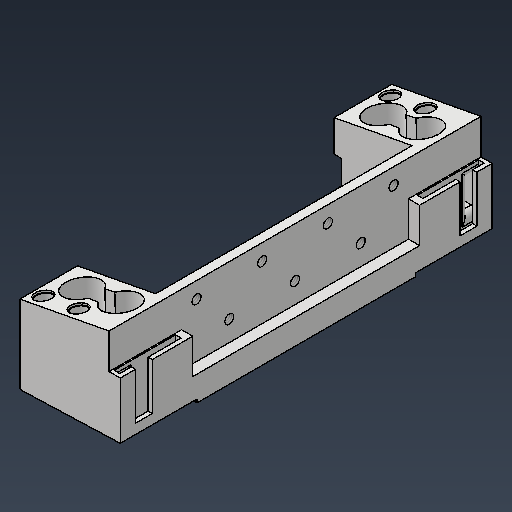
# Autodesk Inventor part: FonrtMount
Saved by Autodesk Inventor 2026.2 (Build 302298010, 298A)
## iProperties
Created: 2026-04-04
Part Number: FonrtMount
Material: Generic
Document SubType Name: Sheet Metal
Designer: szymo
Density: 1 g/cm^3
Appearance: Default
Mass: 17.9089 g
Surface Area: 155.221 cm^2
Volume: 17.9089 cm^3
Sheet Metal Rule: Default
Author: szymo
Autodesk Inventor part; units mm, degrees
(part 1 of 2)
ref_plane "YZ Plane" through (0, 0, 0) normal (1, 0, 0) x (0, 1, 0)
ref_plane "XZ Plane" through (0, 0, 0) normal (0, 1, 0) x (-1, 0, 0)
ref_plane "XY Plane" through (0, 0, 0) normal (0, 0, 1) x (1, 0, 0)
sketch "Sketch1" plane through (0, 0, 0) normal (0, 0, 1) x (1, 0, 0)
  line L0 (-27, 86.2958) -> (-6.5, 86.2958) projected
  line L1 (-6.5, 86.2958) -> (-6.5, 69.7958) projected
  line L2 (-27, 69.7958) -> (-6.5, 69.7958) projected
  line L3 (-27, 86.2958) -> (-27, 69.7958) projected
  line L4 (0, 97) -> (0, 81.9) projected
  line L5 (0, 81.9) -> (-2, 81.9) projected
  line L6 (-4, 93) -> (0, 97) projected
  circle A0 centre (-14.5, 55.2958) radius 14.5 projected
  line L7 (-5.9811, 90.2856) -> (-6, 90.2856)
  line L8 (-6, 90.2856) -> (-6, 69.2958)
  line L9 (-6, 69.2958) -> (-10.7251, 69.2958)
  line L10 (-4, 65.2958) -> (0, 65.2958)
  line L11 (0, 65.2958) -> (0, 81.4)
  line L12 (0, 81.4) -> (-3, 81.4)
  line L13 (-3, 81.4) -> (-3, 90.8556)
  line L14 (-6, 90.2856) -> (-5.9811, 90.2856)
  line L15 (-6, 90.2856) -> (-3, 90.8556)
  line L16 (-9.2085, 69.2958) -> (-9.2085, 68.7958)
  arc A1 (-5.2144, 40.6176) -> (-6.571, 40.1714) centre (-4.0302, 34.7325) ccw construction
  arc A2 (-4.9311, 40.2025) -> (-5.2144, 40.6176) centre (-13, 35.0012) ccw construction
  arc A3 (-5.8414, 39.102) -> (-4.9311, 40.2025) centre (-9.9791, 43.4512) ccw construction
  arc A4 (-5.6366, 38.7217) -> (-5.8414, 39.102) centre (-13, 35.0012) ccw construction
  arc A5 (-4.2168, 38.8762) -> (-5.6366, 38.7217) centre (-4.2821, 32.8735) ccw construction
  arc A6 (-4.026, 38.4112) -> (-4.2168, 38.8762) centre (-13, 35.0012) ccw construction
  arc A7 (-5.1452, 37.524) -> (-4.026, 38.4112) centre (-8.2882, 42.6385) ccw construction
  arc A8 (-5.0239, 37.1095) -> (-5.1452, 37.524) centre (-13, 35.0012) ccw construction
  arc A9 (-3.6031, 36.9654) -> (-5.0239, 37.1095) centre (-4.915, 31.1074) ccw construction
  arc A10 (-3.5132, 36.4709) -> (-3.6031, 36.9654) centre (-13, 35.0012) ccw construction
  arc A11 (-4.7923, 35.8358) -> (-3.5132, 36.4709) centre (-6.8033, 41.492) ccw construction
  arc A12 (-4.7599, 35.4051) -> (-4.7923, 35.8358) centre (-13, 35.0012) ccw construction
  arc A13 (-3.4001, 34.9687) -> (-4.7599, 35.4051) centre (-5.9012, 29.5115) ccw construction
  arc A14 (-3.4149, 34.4663) -> (-3.4001, 34.9687) centre (-13, 35.0012) ccw construction
  arc A15 (-4.7982, 34.1111) -> (-3.4149, 34.4663) centre (-5.5892, 40.0618) ccw construction
  arc A16 (-4.856, 33.6831) -> (-4.7982, 34.1111) centre (-13, 35.0012) ccw construction
  arc A17 (-3.6166, 32.9735) -> (-4.856, 33.6831) centre (-7.1977, 28.1556) ccw construction
  arc A18 (-3.7356, 32.4852) -> (-3.6166, 32.9735) centre (-13, 35.0012) ccw construction
  arc A19 (-5.1625, 32.4253) -> (-3.7356, 32.4852) centre (-4.699, 38.4104) ccw construction
  arc A20 (-5.308, 32.0186) -> (-5.1625, 32.4253) centre (-13, 35.0012) ccw construction
  arc A21 (-4.2432, 31.0669) -> (-5.308, 32.0186) centre (-8.7478, 27.0988) ccw construction
  arc A22 (-4.4611, 30.614) -> (-4.2432, 31.0669) centre (-13, 35.0012) ccw construction
  arc A23 (-5.8693, 30.8521) -> (-4.4611, 30.614) centre (-4.1716, 36.61) ccw construction
  arc A24 (-6.0962, 30.4845) -> (-5.8693, 30.8521) centre (-13, 35.0012) ccw construction
  arc A25 (-5.2526, 29.3322) -> (-6.0962, 30.4845) centre (-10.4837, 26.3874) ccw construction
  arc A26 (-5.5599, 28.9345) -> (-5.2526, 29.3322) centre (-13, 35.0012) ccw construction
  arc A27 (-6.8878, 29.4602) -> (-5.5599, 28.9345) centre (-4.03, 34.7394) ccw construction
  arc A28 (-7.1861, 29.1479) -> (-6.8878, 29.4602) centre (-13, 35.0012) ccw construction
  arc A29 (-6.6005, 27.8453) -> (-7.1861, 29.1479) centre (-12.3296, 26.0525) ccw construction
  arc A30 (-6.9838, 27.5202) -> (-6.6005, 27.8453) centre (-13, 35.0012) ccw construction
  arc A31 (-8.1734, 28.3104) -> (-6.9838, 27.5202) centre (-4.2805, 32.8801) ccw construction
  arc A32 (-8.5302, 28.067) -> (-8.1734, 28.3104) centre (-13, 35.0012) ccw construction
  arc A33 (-8.2282, 26.6712) -> (-8.5302, 28.067) centre (-14.2048, 26.1086) ccw construction
  arc A34 (-8.6707, 26.4328) -> (-8.2282, 26.6712) centre (-13, 35.0012) ccw construction
  arc A35 (-9.6699, 27.4531) -> (-8.6707, 26.4328) centre (-4.912, 31.1136) ccw construction
  arc A36 (-10.0695, 27.2892) -> (-9.6699, 27.4531) centre (-13, 35.0012) ccw construction
  arc A37 (-10.0643, 25.8611) -> (-10.0695, 27.2892) centre (-16.0273, 26.5534) ccw construction
  arc A38 (-10.5467, 25.72) -> (-10.0643, 25.8611) centre (-13, 35.0012) ccw construction
  arc A39 (-11.312, 26.9257) -> (-10.5467, 25.72) centre (-5.897, 29.5169) ccw construction
  arc A40 (-11.737, 26.8485) -> (-11.312, 26.9257) centre (-13, 35.0012) ccw construction
  arc A41 (-12.0288, 25.4504) -> (-11.737, 26.8485) centre (-17.7176, 27.3675) ccw construction
  arc A42 (-12.53, 25.4127) -> (-12.0288, 25.4504) centre (-13, 35.0012) ccw construction
  arc A43 (-13.0279, 26.7512) -> (-12.53, 25.4127) centre (-7.1925, 28.16) ccw construction
  arc A44 (-13.4596, 26.764) -> (-13.0279, 26.7512) centre (-13, 35.0012) ccw construction
  arc A45 (-14.0358, 25.4572) -> (-13.4596, 26.764) centre (-19.2016, 28.5151) ccw construction
  arc A46 (-14.5338, 25.5245) -> (-14.0358, 25.4572) centre (-13, 35.0012) ccw construction
  arc A47 (-14.7426, 26.9373) -> (-14.5338, 25.5245) centre (-8.7418, 27.102) ccw construction
  arc A48 (-15.1622, 27.0396) -> (-14.7426, 26.9373) centre (-13, 35.0012) ccw construction
  arc A49 (-15.9974, 25.8811) -> (-15.1622, 27.0396) centre (-20.4146, 29.9462) ccw construction
  arc A50 (-16.4706, 26.0505) -> (-15.9974, 25.8811) centre (-13, 35.0012) ccw construction
  arc A51 (-16.3811, 27.4758) -> (-16.4706, 26.0505) centre (-10.4772, 26.3893) ccw construction
  arc A52 (-16.7703, 27.6631) -> (-16.3811, 27.4758) centre (-13, 35.0012) ccw construction
  arc A53 (-17.8281, 26.7036) -> (-16.7703, 27.6631) centre (-21.3036, 31.5983) ccw construction
  arc A54 (-18.2557, 26.9677) -> (-17.8281, 26.7036) centre (-13, 35.0012) ccw construction
  arc A55 (-17.8718, 28.3432) -> (-18.2557, 26.9677) centre (-12.3228, 26.053) ccw construction
  arc A56 (-18.2136, 28.6073) -> (-17.8718, 28.3432) centre (-13, 35.0012) ccw construction
  arc A57 (-19.4477, 27.8888) -> (-18.2136, 28.6073) centre (-21.8296, 33.3991) ccw construction
  arc A58 (-19.8111, 28.236) -> (-19.4477, 27.8888) centre (-13, 35.0012) ccw construction
  arc A59 (-19.1496, 29.5016) -> (-19.8111, 28.236) centre (-14.198, 26.1077) ccw construction
  arc A60 (-19.429, 29.831) -> (-19.1496, 29.5016) centre (-13, 35.0012) ccw construction
  arc A61 (-20.7856, 29.3848) -> (-19.429, 29.831) centre (-21.9698, 35.2699) ccw construction
  arc A62 (-21.0689, 29.7999) -> (-20.7856, 29.3848) centre (-13, 35.0012) ccw construction
  arc A63 (-20.1586, 30.9004) -> (-21.0689, 29.7999) centre (-16.0209, 26.5512) ccw construction
  arc A64 (-20.3634, 31.2807) -> (-20.1586, 30.9004) centre (-13, 35.0012) ccw construction
  arc A65 (-21.7832, 31.1262) -> (-20.3634, 31.2807) centre (-21.7179, 37.1289) ccw construction
  arc A66 (-21.974, 31.5912) -> (-21.7832, 31.1262) centre (-13, 35.0012) ccw construction
  arc A67 (-20.8548, 32.4784) -> (-21.974, 31.5912) centre (-17.7118, 27.3639) ccw construction
  arc A68 (-20.9761, 32.8929) -> (-20.8548, 32.4784) centre (-13, 35.0012) ccw construction
  arc A69 (-22.3969, 33.037) -> (-20.9761, 32.8929) centre (-21.085, 38.895) ccw construction
  arc A70 (-22.4868, 33.5315) -> (-22.3969, 33.037) centre (-13, 35.0012) ccw construction
  arc A71 (-21.2077, 34.1666) -> (-22.4868, 33.5315) centre (-19.1967, 28.5104) ccw construction
  arc A72 (-21.2401, 34.5973) -> (-21.2077, 34.1666) centre (-13, 35.0012) ccw construction
  arc A73 (-22.5999, 35.0337) -> (-21.2401, 34.5973) centre (-20.0988, 40.4909) ccw construction
  arc A74 (-22.5851, 35.5361) -> (-22.5999, 35.0337) centre (-13, 35.0012) ccw construction
  arc A75 (-21.2018, 35.8913) -> (-22.5851, 35.5361) centre (-20.4108, 29.9406) ccw construction
  arc A76 (-21.144, 36.3193) -> (-21.2018, 35.8913) centre (-13, 35.0012) ccw construction
  arc A77 (-22.3834, 37.0289) -> (-21.144, 36.3193) centre (-18.8023, 41.8468) ccw construction
  arc A78 (-22.2644, 37.5172) -> (-22.3834, 37.0289) centre (-13, 35.0012) ccw construction
  arc A79 (-20.8375, 37.5771) -> (-22.2644, 37.5172) centre (-21.301, 31.592) ccw construction
  arc A80 (-20.692, 37.9838) -> (-20.8375, 37.5771) centre (-13, 35.0012) ccw construction
  arc A81 (-21.7568, 38.9355) -> (-20.692, 37.9838) centre (-17.2522, 42.9036) ccw construction
  arc A82 (-21.5389, 39.3884) -> (-21.7568, 38.9355) centre (-13, 35.0012) ccw construction
  arc A83 (-20.1307, 39.1503) -> (-21.5389, 39.3884) centre (-21.8284, 33.3924) ccw construction
  arc A84 (-19.9038, 39.5178) -> (-20.1307, 39.1503) centre (-13, 35.0012) ccw construction
  arc A85 (-20.7474, 40.6702) -> (-19.9038, 39.5178) centre (-15.5163, 43.615) ccw construction
  arc A86 (-20.4401, 41.0679) -> (-20.7474, 40.6702) centre (-13, 35.0012) ccw construction
  arc A87 (-19.1122, 40.5422) -> (-20.4401, 41.0679) centre (-21.97, 35.263) ccw construction
  arc A88 (-18.8139, 40.8545) -> (-19.1122, 40.5422) centre (-13, 35.0012) ccw construction
  arc A89 (-19.3995, 42.1571) -> (-18.8139, 40.8545) centre (-13.6704, 43.9499) ccw construction
  arc A90 (-19.0162, 42.4822) -> (-19.3995, 42.1571) centre (-13, 35.0012) ccw construction
  arc A91 (-17.8266, 41.692) -> (-19.0162, 42.4822) centre (-21.7195, 37.1223) ccw construction
  arc A92 (-17.4698, 41.9354) -> (-17.8266, 41.692) centre (-13, 35.0012) ccw construction
  arc A93 (-17.7718, 43.3312) -> (-17.4698, 41.9354) centre (-11.7952, 43.8938) ccw construction
  arc A94 (-17.3293, 43.5696) -> (-17.7718, 43.3312) centre (-13, 35.0012) ccw construction
  arc A95 (-16.3301, 42.5493) -> (-17.3293, 43.5696) centre (-21.088, 38.8888) ccw construction
  arc A96 (-15.9305, 42.7132) -> (-16.3301, 42.5493) centre (-13, 35.0012) ccw construction
  arc A97 (-15.9357, 44.1413) -> (-15.9305, 42.7132) centre (-9.9727, 43.4489) ccw construction
  arc A98 (-15.4533, 44.2824) -> (-15.9357, 44.1413) centre (-13, 35.0012) ccw construction
  arc A99 (-14.688, 43.0767) -> (-15.4533, 44.2824) centre (-20.103, 40.4855) ccw construction
  arc A100 (-14.263, 43.1539) -> (-14.688, 43.0767) centre (-13, 35.0012) ccw construction
  arc A101 (-13.9712, 44.5519) -> (-14.263, 43.1539) centre (-8.2824, 42.6349) ccw construction
  arc A102 (-13.47, 44.5897) -> (-13.9712, 44.5519) centre (-13, 35.0012) ccw construction
  arc A103 (-12.9721, 43.2512) -> (-13.47, 44.5897) centre (-18.8075, 41.8424) ccw construction
  arc A104 (-12.5404, 43.2384) -> (-12.9721, 43.2512) centre (-13, 35.0012) ccw construction
  arc A105 (-11.9642, 44.5452) -> (-12.5404, 43.2384) centre (-6.7984, 41.4873) ccw construction
  arc A106 (-11.4662, 44.4779) -> (-11.9642, 44.5452) centre (-13, 35.0012) ccw construction
  arc A107 (-11.2574, 43.0651) -> (-11.4662, 44.4779) centre (-17.2582, 42.9004) ccw construction
  arc A108 (-10.8378, 42.9628) -> (-11.2574, 43.0651) centre (-13, 35.0012) ccw construction
  arc A109 (-10.0026, 44.1213) -> (-10.8378, 42.9628) centre (-5.5854, 40.0562) ccw construction
  arc A110 (-9.5294, 43.9519) -> (-10.0026, 44.1213) centre (-13, 35.0012) ccw construction
  arc A111 (-9.6189, 42.5266) -> (-9.5294, 43.9519) centre (-15.5228, 43.6131) ccw construction
  arc A112 (-9.2297, 42.3393) -> (-9.6189, 42.5266) centre (-13, 35.0012) ccw construction
  arc A113 (-8.1719, 43.2988) -> (-9.2297, 42.3393) centre (-4.6964, 38.4041) ccw construction
  arc A114 (-7.7443, 43.0347) -> (-8.1719, 43.2988) centre (-13, 35.0012) ccw construction
  arc A115 (-8.1282, 41.6591) -> (-7.7443, 43.0347) centre (-13.6772, 43.9494) ccw construction
  arc A116 (-7.7864, 41.3951) -> (-8.1282, 41.6591) centre (-13, 35.0012) ccw construction
  arc A117 (-6.5523, 42.1136) -> (-7.7864, 41.3951) centre (-4.1704, 36.6033) ccw construction
  arc A118 (-6.1889, 41.7664) -> (-6.5523, 42.1136) centre (-13, 35.0012) ccw construction
  arc A119 (-6.8504, 40.5008) -> (-6.1889, 41.7664) centre (-11.802, 43.8947) ccw construction
  arc A120 (-6.571, 40.1714) -> (-6.8504, 40.5008) centre (-13, 35.0012) ccw construction
  circle A121 centre (-13, 35.0012) radius 9.6 construction
  line L17 (-4, 65.2958) -> (-27, 65.2958)
  line L18 (-27, 65.2958) -> (-27, 24.2538) construction
  line L19 (-27, 65.2958) -> (-27, 69.2958)
  line L20 (-27, 69.2958) -> (-9.2085, 69.2958)
  line L21 (-3.3867, 91.8) -> (-29.4, 86.8578)
  line L22 (-29.4, 86.8578) -> (-29.2133, 85.8753)
  line L23 (-29.2133, 85.8753) -> (-3.2, 90.8176)
  line L24 (-3.3867, 91.8) -> (-3.2, 90.8176)
  line L25 (0, 97) -> (0, 84.632) projected
  line L26 (-3, 84.632) -> (-3, 92) projected
  line L27 (-5, 92) -> (0, 97) projected
  line L28 (-29.4, 86.8578) -> (-29.4, 73.8558) construction
  line L29 (-3, 92) -> (-5, 92) projected
  line L30 (-3, 84.632) -> (0, 84.632) projected
  point P0 (-25, 65.2958)
  point P1 (-18.2749, 69.2958)
  point P2 (-3, 46.4641)
  point P3 (-6, 43.5485)
  point P4 (-6, 67.0432)
  point P5 (-6, 65.2958)
  point P6 (-3, 64.1276)
  point P7 (-3, 65.2958)
  dimension "d0" = 4.5
  dimension "d1" = 0.5
  dimension "d2" = 0.5
  dimension "d6" = 0.5
  dimension "d11" = 0.5
  dimension "d32" = 2
  dimension "d140" = 0
  dimension "d142" = 1
  dimension "d157" = 0
  dimension "d164" = 0
  dimension "d168" = 79.243
  dimension "d169" = 0.2
  dimension "d170" = 0.4
  dimension "d172" = 0.2
  constraints: 38 end point, 7 perpendicular, 4 vertical, 3 horizontal, 3 point on circle, 2 collinear, 1 coincident, 1 parallel, 1 point on line, 1 tangent, 3 other
  measures "d0" distance between parallel lines of L10 L2
  measures "d1" distance between parallel lines of L2 L9
  measures "d2" distance between parallel lines of L1 L8
  measures "d6" distance between parallel lines of L5 L12
  measures "d11" distance of L16.start L16.end
  measures "d32" distance edge to line of A0 L18
  measures "d140" distance from line of L23 L0.start
  measures "d142" distance between parallel lines of L21 L23
  measures "d157" distance between parallel lines of L23 L15
  measures "d164" distance between parallel lines of L26 L13
  measures "d168" angle of L23 L8
  measures "d169" distance from line of L26 L23.end
  measures "d170" distance edge to line of A0 L28
  measures "d172" distance from line of L29 L21.start
extrude "Extrusion2" add sketch "Sketch1" along normal blind 19.75 and the other way blind 17.65 contours L15 L13 L12 L11 L10 A0 L16 L9 L8
sketch "Sketch2" plane through (0, 0, -17.65) normal (0, 0, -1) x (-1, 0, 0)
  arc A0 (6.571, 40.1714) -> (5.2144, 40.6176) centre (4.0302, 34.7325) ccw construction
  arc A1 (5.2144, 40.6176) -> (4.9311, 40.2025) centre (13, 35.0012) ccw construction
  arc A2 (4.9311, 40.2025) -> (5.8414, 39.102) centre (9.9791, 43.4512) ccw construction
  arc A3 (5.8414, 39.102) -> (5.6366, 38.7217) centre (13, 35.0012) ccw construction
  arc A4 (5.6366, 38.7217) -> (4.2168, 38.8762) centre (4.2821, 32.8735) ccw construction
  arc A5 (4.2168, 38.8762) -> (4.026, 38.4112) centre (13, 35.0012) ccw construction
  arc A6 (4.026, 38.4112) -> (5.1452, 37.524) centre (8.2882, 42.6385) ccw construction
  arc A7 (5.1452, 37.524) -> (5.0239, 37.1095) centre (13, 35.0012) ccw construction
  arc A8 (5.0239, 37.1095) -> (3.6031, 36.9654) centre (4.915, 31.1074) ccw construction
  arc A9 (3.6031, 36.9654) -> (3.5132, 36.4709) centre (13, 35.0012) ccw construction
  arc A10 (3.5132, 36.4709) -> (4.7923, 35.8358) centre (6.8033, 41.492) ccw construction
  arc A11 (4.7923, 35.8358) -> (4.7599, 35.4051) centre (13, 35.0012) ccw construction
  arc A12 (4.7599, 35.4051) -> (3.4001, 34.9687) centre (5.9012, 29.5115) ccw construction
  arc A13 (3.4001, 34.9687) -> (3.4149, 34.4663) centre (13, 35.0012) ccw construction
  arc A14 (3.4149, 34.4663) -> (4.7982, 34.1111) centre (5.5892, 40.0618) ccw construction
  arc A15 (4.7982, 34.1111) -> (4.856, 33.6831) centre (13, 35.0012) ccw construction
  arc A16 (4.856, 33.6831) -> (3.6166, 32.9735) centre (7.1977, 28.1556) ccw construction
  arc A17 (3.6166, 32.9735) -> (3.7356, 32.4852) centre (13, 35.0012) ccw construction
  arc A18 (3.7356, 32.4852) -> (5.1625, 32.4253) centre (4.699, 38.4104) ccw construction
  arc A19 (5.1625, 32.4253) -> (5.308, 32.0186) centre (13, 35.0012) ccw construction
  arc A20 (5.308, 32.0186) -> (4.2432, 31.0669) centre (8.7478, 27.0988) ccw construction
  arc A21 (4.2432, 31.0669) -> (4.4611, 30.614) centre (13, 35.0012) ccw construction
  arc A22 (4.4611, 30.614) -> (5.8693, 30.8521) centre (4.1716, 36.61) ccw construction
  arc A23 (5.8693, 30.8521) -> (6.0962, 30.4845) centre (13, 35.0012) ccw construction
  arc A24 (6.0962, 30.4845) -> (5.2526, 29.3322) centre (10.4837, 26.3874) ccw construction
  arc A25 (5.2526, 29.3322) -> (5.5599, 28.9345) centre (13, 35.0012) ccw construction
  arc A26 (5.5599, 28.9345) -> (6.8878, 29.4602) centre (4.03, 34.7394) ccw construction
  arc A27 (6.8878, 29.4602) -> (7.1861, 29.1479) centre (13, 35.0012) ccw construction
  arc A28 (7.1861, 29.1479) -> (6.6005, 27.8453) centre (12.3296, 26.0525) ccw construction
  arc A29 (6.6005, 27.8453) -> (6.9838, 27.5202) centre (13, 35.0012) ccw construction
  arc A30 (6.9838, 27.5202) -> (8.1734, 28.3104) centre (4.2805, 32.8801) ccw construction
  arc A31 (8.1734, 28.3104) -> (8.5302, 28.067) centre (13, 35.0012) ccw construction
  arc A32 (8.5302, 28.067) -> (8.2282, 26.6712) centre (14.2048, 26.1086) ccw construction
  arc A33 (8.2282, 26.6712) -> (8.6707, 26.4328) centre (13, 35.0012) ccw construction
  arc A34 (8.6707, 26.4328) -> (9.6699, 27.4531) centre (4.912, 31.1136) ccw construction
  arc A35 (9.6699, 27.4531) -> (10.0695, 27.2892) centre (13, 35.0012) ccw construction
  arc A36 (10.0695, 27.2892) -> (10.0643, 25.8611) centre (16.0273, 26.5534) ccw construction
  arc A37 (10.0643, 25.8611) -> (10.5467, 25.72) centre (13, 35.0012) ccw construction
  arc A38 (10.5467, 25.72) -> (11.312, 26.9257) centre (5.897, 29.5169) ccw construction
  arc A39 (11.312, 26.9257) -> (11.737, 26.8485) centre (13, 35.0012) ccw construction
  arc A40 (11.737, 26.8485) -> (12.0288, 25.4504) centre (17.7176, 27.3675) ccw construction
  arc A41 (12.0288, 25.4504) -> (12.53, 25.4127) centre (13, 35.0012) ccw construction
  arc A42 (12.53, 25.4127) -> (13.0279, 26.7512) centre (7.1925, 28.16) ccw construction
  arc A43 (13.0279, 26.7512) -> (13.4596, 26.764) centre (13, 35.0012) ccw construction
  arc A44 (13.4596, 26.764) -> (14.0358, 25.4572) centre (19.2016, 28.5151) ccw construction
  arc A45 (14.0358, 25.4572) -> (14.5338, 25.5245) centre (13, 35.0012) ccw construction
  arc A46 (14.5338, 25.5245) -> (14.7426, 26.9373) centre (8.7418, 27.102) ccw construction
  arc A47 (14.7426, 26.9373) -> (15.1622, 27.0396) centre (13, 35.0012) ccw construction
  arc A48 (15.1622, 27.0396) -> (15.9974, 25.8811) centre (20.4146, 29.9462) ccw construction
  arc A49 (15.9974, 25.8811) -> (16.4706, 26.0505) centre (13, 35.0012) ccw construction
  arc A50 (16.4706, 26.0505) -> (16.3811, 27.4758) centre (10.4772, 26.3893) ccw construction
  arc A51 (16.3811, 27.4758) -> (16.7703, 27.6631) centre (13, 35.0012) ccw construction
  arc A52 (16.7703, 27.6631) -> (17.8281, 26.7036) centre (21.3036, 31.5983) ccw construction
  arc A53 (17.8281, 26.7036) -> (18.2557, 26.9677) centre (13, 35.0012) ccw construction
  arc A54 (18.2557, 26.9677) -> (17.8718, 28.3432) centre (12.3228, 26.053) ccw construction
  arc A55 (17.8718, 28.3432) -> (18.2136, 28.6073) centre (13, 35.0012) ccw construction
  arc A56 (18.2136, 28.6073) -> (19.4477, 27.8888) centre (21.8296, 33.3991) ccw construction
  arc A57 (19.4477, 27.8888) -> (19.8111, 28.236) centre (13, 35.0012) ccw construction
  arc A58 (19.8111, 28.236) -> (19.1496, 29.5016) centre (14.198, 26.1077) ccw construction
  arc A59 (19.1496, 29.5016) -> (19.429, 29.831) centre (13, 35.0012) ccw construction
  arc A60 (19.429, 29.831) -> (20.7856, 29.3848) centre (21.9698, 35.2699) ccw construction
  arc A61 (20.7856, 29.3848) -> (21.0689, 29.7999) centre (13, 35.0012) ccw construction
  arc A62 (21.0689, 29.7999) -> (20.1586, 30.9004) centre (16.0209, 26.5512) ccw construction
  arc A63 (20.1586, 30.9004) -> (20.3634, 31.2807) centre (13, 35.0012) ccw construction
  arc A64 (20.3634, 31.2807) -> (21.7832, 31.1262) centre (21.7179, 37.1289) ccw construction
  arc A65 (21.7832, 31.1262) -> (21.974, 31.5912) centre (13, 35.0012) ccw construction
  arc A66 (21.974, 31.5912) -> (20.8548, 32.4784) centre (17.7118, 27.3639) ccw construction
  arc A67 (20.8548, 32.4784) -> (20.9761, 32.8929) centre (13, 35.0012) ccw construction
  arc A68 (20.9761, 32.8929) -> (22.3969, 33.037) centre (21.085, 38.895) ccw construction
  arc A69 (22.3969, 33.037) -> (22.4868, 33.5315) centre (13, 35.0012) ccw construction
  arc A70 (22.4868, 33.5315) -> (21.2077, 34.1666) centre (19.1967, 28.5104) ccw construction
  arc A71 (21.2077, 34.1666) -> (21.2401, 34.5973) centre (13, 35.0012) ccw construction
  arc A72 (21.2401, 34.5973) -> (22.5999, 35.0337) centre (20.0988, 40.4909) ccw construction
  arc A73 (22.5999, 35.0337) -> (22.5851, 35.5361) centre (13, 35.0012) ccw construction
  arc A74 (22.5851, 35.5361) -> (21.2018, 35.8913) centre (20.4108, 29.9406) ccw construction
  arc A75 (21.2018, 35.8913) -> (21.144, 36.3193) centre (13, 35.0012) ccw construction
  arc A76 (21.144, 36.3193) -> (22.3834, 37.0289) centre (18.8023, 41.8468) ccw construction
  arc A77 (22.3834, 37.0289) -> (22.2644, 37.5172) centre (13, 35.0012) ccw construction
  arc A78 (22.2644, 37.5172) -> (20.8375, 37.5771) centre (21.301, 31.592) ccw construction
  arc A79 (20.8375, 37.5771) -> (20.692, 37.9838) centre (13, 35.0012) ccw construction
  arc A80 (20.692, 37.9838) -> (21.7568, 38.9355) centre (17.2522, 42.9036) ccw construction
  arc A81 (21.7568, 38.9355) -> (21.5389, 39.3884) centre (13, 35.0012) ccw construction
  arc A82 (21.5389, 39.3884) -> (20.1307, 39.1503) centre (21.8284, 33.3924) ccw construction
  arc A83 (20.1307, 39.1503) -> (19.9038, 39.5178) centre (13, 35.0012) ccw construction
  arc A84 (19.9038, 39.5178) -> (20.7474, 40.6702) centre (15.5163, 43.615) ccw construction
  arc A85 (20.7474, 40.6702) -> (20.4401, 41.0679) centre (13, 35.0012) ccw construction
  arc A86 (20.4401, 41.0679) -> (19.1122, 40.5422) centre (21.97, 35.263) ccw construction
  arc A87 (19.1122, 40.5422) -> (18.8139, 40.8545) centre (13, 35.0012) ccw construction
  arc A88 (18.8139, 40.8545) -> (19.3995, 42.1571) centre (13.6704, 43.9499) ccw construction
  arc A89 (19.3995, 42.1571) -> (19.0162, 42.4822) centre (13, 35.0012) ccw construction
  arc A90 (19.0162, 42.4822) -> (17.8266, 41.692) centre (21.7195, 37.1223) ccw construction
  arc A91 (17.8266, 41.692) -> (17.4698, 41.9354) centre (13, 35.0012) ccw construction
  arc A92 (17.4698, 41.9354) -> (17.7718, 43.3312) centre (11.7952, 43.8938) ccw construction
  arc A93 (17.7718, 43.3312) -> (17.3293, 43.5696) centre (13, 35.0012) ccw construction
  arc A94 (17.3293, 43.5696) -> (16.3301, 42.5493) centre (21.088, 38.8888) ccw construction
  arc A95 (16.3301, 42.5493) -> (15.9305, 42.7132) centre (13, 35.0012) ccw construction
  arc A96 (15.9305, 42.7132) -> (15.9357, 44.1413) centre (9.9727, 43.4489) ccw construction
  arc A97 (15.9357, 44.1413) -> (15.4533, 44.2824) centre (13, 35.0012) ccw construction
  arc A98 (15.4533, 44.2824) -> (14.688, 43.0767) centre (20.103, 40.4855) ccw construction
  arc A99 (14.688, 43.0767) -> (14.263, 43.1539) centre (13, 35.0012) ccw construction
  arc A100 (14.263, 43.1539) -> (13.9712, 44.5519) centre (8.2824, 42.6349) ccw construction
  arc A101 (13.9712, 44.5519) -> (13.47, 44.5897) centre (13, 35.0012) ccw construction
  arc A102 (13.47, 44.5897) -> (12.9721, 43.2512) centre (18.8075, 41.8424) ccw construction
  arc A103 (12.9721, 43.2512) -> (12.5404, 43.2384) centre (13, 35.0012) ccw construction
  arc A104 (12.5404, 43.2384) -> (11.9642, 44.5452) centre (6.7984, 41.4873) ccw construction
  arc A105 (11.9642, 44.5452) -> (11.4662, 44.4779) centre (13, 35.0012) ccw construction
  arc A106 (11.4662, 44.4779) -> (11.2574, 43.0651) centre (17.2582, 42.9004) ccw construction
  arc A107 (11.2574, 43.0651) -> (10.8378, 42.9628) centre (13, 35.0012) ccw construction
  arc A108 (10.8378, 42.9628) -> (10.0026, 44.1213) centre (5.5854, 40.0562) ccw construction
  arc A109 (10.0026, 44.1213) -> (9.5294, 43.9519) centre (13, 35.0012) ccw construction
  arc A110 (9.5294, 43.9519) -> (9.6189, 42.5266) centre (15.5228, 43.6131) ccw construction
  arc A111 (9.6189, 42.5266) -> (9.2297, 42.3393) centre (13, 35.0012) ccw construction
  arc A112 (9.2297, 42.3393) -> (8.1719, 43.2988) centre (4.6964, 38.4041) ccw construction
  arc A113 (8.1719, 43.2988) -> (7.7443, 43.0347) centre (13, 35.0012) ccw construction
  arc A114 (7.7443, 43.0347) -> (8.1282, 41.6591) centre (13.6772, 43.9494) ccw construction
  arc A115 (8.1282, 41.6591) -> (7.7864, 41.3951) centre (13, 35.0012) ccw construction
  arc A116 (7.7864, 41.3951) -> (6.5523, 42.1136) centre (4.1704, 36.6033) ccw construction
  arc A117 (6.5523, 42.1136) -> (6.1889, 41.7664) centre (13, 35.0012) ccw construction
  arc A118 (6.1889, 41.7664) -> (6.8504, 40.5008) centre (11.802, 43.8947) ccw construction
  arc A119 (6.8504, 40.5008) -> (6.571, 40.1714) centre (13, 35.0012) ccw construction
  circle A120 centre (13, 35.0012) radius 9.6 construction
  line L0 (23.8, 32.6031) -> (23.8, 65.2958) construction
  line L1 (9.2085, 69.2958) -> (6, 69.2958) projected
  line L2 (6, 69.2958) -> (6, 90.2856) projected
  line L3 (6, 90.2856) -> (3, 90.8556) projected
  line L4 (3, 90.8556) -> (3, 81.4) projected
  line L5 (3, 81.4) -> (0, 81.4) projected
  line L6 (0, 81.4) -> (0, 65.2958) projected
  line L7 (0, 65.2958) -> (4, 65.2958) projected
  line L8 (4, 65.2958) -> (23.8, 65.2958)
  line L9 (23.8, 65.2958) -> (23.8, 69.2958)
  line L10 (23.8, 69.2958) -> (9.2085, 69.2958)
  circle A121 centre (14.5, 55.2958) radius 14.5 projected
  arc A122 (9.2085, 68.7958) -> (4, 65.2958) centre (14.5, 55.2958) ccw projected
  line L11 (9.2085, 68.7958) -> (9.2085, 69.2958) projected
  point P0 (0, 0)
  point P1 (9.2085, 69.2958)
  point P2 (9.2085, 69.2958)
  dimension "d33" = 5.2
  dimension "d35" = 1.2
  dimension "d175" = 0.5
  dimension "d176" = 4.5
  constraints: 8 end point, 2 vertical, 1 coincident, 1 horizontal, 1 perpendicular, 3 other
  measures "d33" distance edge to line of A121 L0
  measures "d175" distance edge to line of A121 L10
  measures "d176" distance edge to line of A121 L8
extrude "Extrusion3" add sketch "Sketch2" along normal blind 16.85 contours L11 A121 L7 L6 L5 L4 L3 L2 L1 | L10 A121 L11 | L10 A121 L9 L8 | L10 L9 A121
sketch "Sketch3" plane through (0, 0, 19.75) normal (0, 0, 1) x (1, 0, 0)
  arc A0 (-20.6322, 38.1335) -> (-22.0597, 38.1763) centre (-21.5245, 32.1971) ccw construction
  arc A1 (-22.0597, 38.1763) -> (-22.2135, 37.6978) centre (-13, 35.0012) ccw construction
  arc A2 (-22.2135, 37.6978) -> (-21.0283, 36.901) centre (-18.2955, 42.246) ccw construction
  arc A3 (-21.0283, 36.901) -> (-21.1167, 36.4782) centre (-13, 35.0012) ccw construction
  arc A4 (-21.1167, 36.4782) -> (-22.5219, 36.2233) centre (-20.7552, 30.4861) ccw construction
  arc A5 (-22.5219, 36.2233) -> (-22.5728, 35.7233) centre (-13, 35.0012) ccw construction
  arc A6 (-22.5728, 35.7233) -> (-21.2478, 35.1903) centre (-19.6861, 40.9866) ccw construction
  arc A7 (-21.2478, 35.1903) -> (-21.2464, 34.7584) centre (-13, 35.0012) ccw construction
  arc A8 (-21.2464, 34.7584) -> (-22.5679, 34.2168) centre (-19.647, 28.9724) ccw construction
  arc A9 (-22.5679, 34.2168) -> (-22.5137, 33.7172) centre (-13, 35.0012) ccw construction
  arc A10 (-22.5137, 33.7172) -> (-21.1069, 33.4714) centre (-20.7844, 39.4657) ccw construction
  arc A11 (-21.1069, 33.4714) -> (-21.0157, 33.0492) centre (-13, 35.0012) ccw construction
  arc A12 (-21.0157, 33.0492) -> (-22.1957, 32.2447) centre (-18.2483, 27.7221) ccw construction
  arc A13 (-22.1957, 32.2447) -> (-22.0389, 31.7672) centre (-13, 35.0012) ccw construction
  arc A14 (-22.0389, 31.7672) -> (-20.6117, 31.8193) centre (-21.5425, 37.7497) ccw construction
  arc A15 (-20.6117, 31.8193) -> (-20.4347, 31.4253) centre (-13, 35.0012) ccw construction
  arc A16 (-20.4347, 31.4253) -> (-21.4217, 30.393) centre (-16.6202, 26.79) ccw construction
  arc A17 (-21.4217, 30.393) -> (-21.169, 29.9586) centre (-13, 35.0012) ccw construction
  arc A18 (-21.169, 29.9586) -> (-19.7838, 30.3062) centre (-21.9273, 35.9136) ccw construction
  arc A19 (-19.7838, 30.3062) -> (-19.5288, 29.9576) centre (-13, 35.0012) ccw construction
  arc A20 (-19.5288, 29.9576) -> (-20.2796, 28.7428) centre (-14.8338, 26.2168) ccw construction
  arc A21 (-20.2796, 28.7428) -> (-19.9421, 28.3704) centre (-13, 35.0012) ccw construction
  arc A22 (-19.9421, 28.3704) -> (-18.6594, 28.9984) centre (-21.9219, 34.0375) ccw construction
  arc A23 (-18.6594, 28.9984) -> (-18.3375, 28.7104) centre (-13, 35.0012) ccw construction
  arc A24 (-18.3375, 28.7104) -> (-18.8193, 27.366) centre (-12.9674, 26.0275) ccw construction
  arc A25 (-18.8193, 27.366) -> (-18.4117, 27.0719) centre (-13, 35.0012) ccw construction
  arc A26 (-18.4117, 27.0719) -> (-17.2877, 27.9529) centre (-21.5266, 32.2036) ccw construction
  arc A27 (-17.2877, 27.9529) -> (-16.9129, 27.7382) centre (-13, 35.0012) ccw construction
  arc A28 (-16.9129, 27.7382) -> (-17.1047, 26.323) centre (-11.1024, 26.2303) ccw construction
  arc A29 (-17.1047, 26.323) -> (-16.6449, 26.12) centre (-13, 35.0012) ccw construction
  arc A30 (-16.6449, 26.12) -> (-15.7286, 27.2155) centre (-20.7586, 30.492) ccw construction
  arc A31 (-15.7286, 27.2155) -> (-15.3174, 27.0834) centre (-13, 35.0012) ccw construction
  arc A32 (-15.3174, 27.0834) -> (-15.2107, 25.6592) centre (-9.3203, 26.8165) ccw construction
  arc A33 (-15.2107, 25.6592) -> (-14.7187, 25.5563) centre (-13, 35.0012) ccw construction
  arc A34 (-14.7187, 25.5563) -> (-14.0502, 26.8183) centre (-19.6515, 28.9774) ccw construction
  arc A35 (-14.0502, 26.8183) -> (-13.6205, 26.7746) centre (-13, 35.0012) ccw construction
  arc A36 (-13.6205, 26.7746) -> (-13.2201, 25.4037) centre (-7.699, 27.7605) ccw construction
  arc A37 (-13.2201, 25.4037) -> (-12.7175, 25.4054) centre (-13, 35.0012) ccw construction
  arc A38 (-12.7175, 25.4054) -> (-12.3259, 26.7788) centre (-18.2538, 27.7261) ccw construction
  arc A39 (-12.3259, 26.7788) -> (-11.8965, 26.8253) centre (-13, 35.0012) ccw construction
  arc A40 (-11.8965, 26.8253) -> (-11.2198, 25.5677) centre (-6.3094, 29.0208) ccw construction
  arc A41 (-11.2198, 25.5677) -> (-10.7286, 25.6738) centre (-13, 35.0012) ccw construction
  arc A42 (-10.7286, 25.6738) -> (-10.6311, 27.0986) centre (-16.6264, 26.7928) ccw construction
  arc A43 (-10.6311, 27.0986) -> (-10.2208, 27.2334) centre (-13, 35.0012) ccw construction
  arc A44 (-10.2208, 27.2334) -> (-9.2974, 26.144) centre (-5.2122, 30.5426) ccw construction
  arc A45 (-9.2974, 26.144) -> (-8.8389, 26.3499) centre (-13, 35.0012) ccw construction
  arc A46 (-8.8389, 26.3499) -> (-9.0399, 27.7638) centre (-14.8405, 26.2182) ccw construction
  arc A47 (-9.0399, 27.7638) -> (-8.6665, 27.981) centre (-13, 35.0012) ccw construction
  arc A48 (-8.6665, 27.981) -> (-7.5368, 27.1073) centre (-4.4554, 32.2592) ccw construction
  arc A49 (-7.5368, 27.1073) -> (-7.1311, 27.4041) centre (-13, 35.0012) ccw construction
  arc A50 (-7.1311, 27.4041) -> (-7.6217, 28.7453) centre (-12.9742, 26.0274) ccw construction
  arc A51 (-7.6217, 28.7453) -> (-7.3016, 29.0354) centre (-13, 35.0012) ccw construction
  arc A52 (-7.3016, 29.0354) -> (-6.0149, 28.4157) centre (-4.072, 34.0956) ccw construction
  arc A53 (-6.0149, 28.4157) -> (-5.6799, 28.7903) centre (-13, 35.0012) ccw construction
  arc A54 (-5.6799, 28.7903) -> (-6.4385, 30.0002) centre (-11.109, 26.2289) ccw construction
  arc A55 (-6.4385, 30.0002) -> (-6.1858, 30.3505) centre (-13, 35.0012) ccw construction
  arc A56 (-6.1858, 30.3505) -> (-4.7984, 30.0119) centre (-4.0788, 35.9716) ccw construction
  arc A57 (-4.7984, 30.0119) -> (-4.5485, 30.448) centre (-13, 35.0012) ccw construction
  arc A58 (-4.5485, 30.448) -> (-5.5422, 31.4737) centre (-9.3265, 26.8137) ccw construction
  arc A59 (-5.5422, 31.4737) -> (-5.3678, 31.8689) centre (-13, 35.0012) ccw construction
  arc A60 (-5.3678, 31.8689) -> (-3.9403, 31.8261) centre (-4.4755, 37.8053) ccw construction
  arc A61 (-3.9403, 31.8261) -> (-3.7865, 32.3046) centre (-13, 35.0012) ccw construction
  arc A62 (-3.7865, 32.3046) -> (-4.9717, 33.1014) centre (-7.7045, 27.7564) ccw construction
  arc A63 (-4.9717, 33.1014) -> (-4.8833, 33.5242) centre (-13, 35.0012) ccw construction
  arc A64 (-4.8833, 33.5242) -> (-3.4781, 33.7791) centre (-5.2448, 39.5163) ccw construction
  arc A65 (-3.4781, 33.7791) -> (-3.4272, 34.2791) centre (-13, 35.0012) ccw construction
  arc A66 (-3.4272, 34.2791) -> (-4.7522, 34.8121) centre (-6.3139, 29.0157) ccw construction
  arc A67 (-4.7522, 34.8121) -> (-4.7536, 35.244) centre (-13, 35.0012) ccw construction
  arc A68 (-4.7536, 35.244) -> (-3.4321, 35.7855) centre (-6.353, 41.03) ccw construction
  arc A69 (-3.4321, 35.7855) -> (-3.4863, 36.2852) centre (-13, 35.0012) ccw construction
  arc A70 (-3.4863, 36.2852) -> (-4.8931, 36.531) centre (-5.2156, 30.5367) ccw construction
  arc A71 (-4.8931, 36.531) -> (-4.9843, 36.9532) centre (-13, 35.0012) ccw construction
  arc A72 (-4.9843, 36.9532) -> (-3.8043, 37.7577) centre (-7.7517, 42.2803) ccw construction
  arc A73 (-3.8043, 37.7577) -> (-3.9611, 38.2352) centre (-13, 35.0012) ccw construction
  arc A74 (-3.9611, 38.2352) -> (-5.3883, 38.1831) centre (-4.4575, 32.2527) ccw construction
  arc A75 (-5.3883, 38.1831) -> (-5.5653, 38.5771) centre (-13, 35.0012) ccw construction
  arc A76 (-5.5653, 38.5771) -> (-4.5783, 39.6094) centre (-9.3798, 43.2124) ccw construction
  arc A77 (-4.5783, 39.6094) -> (-4.831, 40.0438) centre (-13, 35.0012) ccw construction
  arc A78 (-4.831, 40.0438) -> (-6.2162, 39.6962) centre (-4.0727, 34.0888) ccw construction
  arc A79 (-6.2162, 39.6962) -> (-6.4712, 40.0448) centre (-13, 35.0012) ccw construction
  arc A80 (-6.4712, 40.0448) -> (-5.7204, 41.2596) centre (-11.1662, 43.7856) ccw construction
  arc A81 (-5.7204, 41.2596) -> (-6.0579, 41.632) centre (-13, 35.0012) ccw construction
  arc A82 (-6.0579, 41.632) -> (-7.3406, 41.004) centre (-4.0781, 35.9649) ccw construction
  arc A83 (-7.3406, 41.004) -> (-7.6625, 41.292) centre (-13, 35.0012) ccw construction
  arc A84 (-7.6625, 41.292) -> (-7.1807, 42.6364) centre (-13.0326, 43.9749) ccw construction
  arc A85 (-7.1807, 42.6364) -> (-7.5883, 42.9305) centre (-13, 35.0012) ccw construction
  arc A86 (-7.5883, 42.9305) -> (-8.7123, 42.0495) centre (-4.4734, 37.7988) ccw construction
  arc A87 (-8.7123, 42.0495) -> (-9.0871, 42.2642) centre (-13, 35.0012) ccw construction
  arc A88 (-9.0871, 42.2642) -> (-8.8953, 43.6794) centre (-14.8976, 43.7721) ccw construction
  arc A89 (-8.8953, 43.6794) -> (-9.3551, 43.8824) centre (-13, 35.0012) ccw construction
  arc A90 (-9.3551, 43.8824) -> (-10.2714, 42.7869) centre (-5.2414, 39.5104) ccw construction
  arc A91 (-10.2714, 42.7869) -> (-10.6826, 42.919) centre (-13, 35.0012) ccw construction
  arc A92 (-10.6826, 42.919) -> (-10.7893, 44.3432) centre (-16.6797, 43.1859) ccw construction
  arc A93 (-10.7893, 44.3432) -> (-11.2813, 44.4461) centre (-13, 35.0012) ccw construction
  arc A94 (-11.2813, 44.4461) -> (-11.9498, 43.1841) centre (-6.3485, 41.025) ccw construction
  arc A95 (-11.9498, 43.1841) -> (-12.3795, 43.2278) centre (-13, 35.0012) ccw construction
  arc A96 (-12.3795, 43.2278) -> (-12.7799, 44.5987) centre (-18.301, 42.2419) ccw construction
  arc A97 (-12.7799, 44.5987) -> (-13.2825, 44.597) centre (-13, 35.0012) ccw construction
  arc A98 (-13.2825, 44.597) -> (-13.6741, 43.2236) centre (-7.7462, 42.2763) ccw construction
  arc A99 (-13.6741, 43.2236) -> (-14.1035, 43.1771) centre (-13, 35.0012) ccw construction
  arc A100 (-14.1035, 43.1771) -> (-14.7802, 44.4347) centre (-19.6906, 40.9816) ccw construction
  arc A101 (-14.7802, 44.4347) -> (-15.2714, 44.3286) centre (-13, 35.0012) ccw construction
  arc A102 (-15.2714, 44.3286) -> (-15.3689, 42.9038) centre (-9.3736, 43.2096) ccw construction
  arc A103 (-15.3689, 42.9038) -> (-15.7792, 42.769) centre (-13, 35.0012) ccw construction
  arc A104 (-15.7792, 42.769) -> (-16.7026, 43.8584) centre (-20.7878, 39.4598) ccw construction
  arc A105 (-16.7026, 43.8584) -> (-17.1611, 43.6525) centre (-13, 35.0012) ccw construction
  arc A106 (-17.1611, 43.6525) -> (-16.9601, 42.2386) centre (-11.1595, 43.7842) ccw construction
  arc A107 (-16.9601, 42.2386) -> (-17.3335, 42.0214) centre (-13, 35.0012) ccw construction
  arc A108 (-17.3335, 42.0214) -> (-18.4632, 42.8951) centre (-21.5446, 37.7432) ccw construction
  arc A109 (-18.4632, 42.8951) -> (-18.8689, 42.5983) centre (-13, 35.0012) ccw construction
  arc A110 (-18.8689, 42.5983) -> (-18.3783, 41.2571) centre (-13.0258, 43.975) ccw construction
  arc A111 (-18.3783, 41.2571) -> (-18.6984, 40.967) centre (-13, 35.0012) ccw construction
  arc A112 (-18.6984, 40.967) -> (-19.9851, 41.5867) centre (-21.928, 35.9068) ccw construction
  arc A113 (-19.9851, 41.5867) -> (-20.3201, 41.2121) centre (-13, 35.0012) ccw construction
  arc A114 (-20.3201, 41.2121) -> (-19.5615, 40.0022) centre (-14.891, 43.7735) ccw construction
  arc A115 (-19.5615, 40.0022) -> (-19.8142, 39.6519) centre (-13, 35.0012) ccw construction
  arc A116 (-19.8142, 39.6519) -> (-21.2016, 39.9905) centre (-21.9212, 34.0308) ccw construction
  arc A117 (-21.2016, 39.9905) -> (-21.4515, 39.5544) centre (-13, 35.0012) ccw construction
  arc A118 (-21.4515, 39.5544) -> (-20.4578, 38.5287) centre (-16.6735, 43.1886) ccw construction
  arc A119 (-20.4578, 38.5287) -> (-20.6322, 38.1335) centre (-13, 35.0012) ccw construction
  line L0 (-6, 69.2958) -> (-9.2085, 69.2958) projected
  line L1 (-4, 65.2958) -> (0, 65.2958) projected
  line L2 (0, 65.2958) -> (0, 81.4) projected
  line L3 (0, 81.4) -> (-3, 81.4) projected
  line L4 (-3, 81.4) -> (-3, 90.8556) projected
  line L5 (-3, 90.8556) -> (-6, 90.2856) projected
  line L6 (-6, 90.2856) -> (-6, 69.2958) projected
  circle A120 centre (-13, 35.0012) radius 9.6
  line L7 (-23.8, 30.4052) -> (-23.8, 69.2958)
  line L8 (-23.8, 69.2958) -> (-9.2085, 69.2958)
  line L9 (-4, 65.2958) -> (-23.8, 65.2958)
  line L10 (-4, 65.2958) -> (-23.8, 65.2958)
  circle A121 centre (-14.5, 55.2958) radius 14.5 projected
  arc A122 (-4, 65.2958) -> (-9.2085, 68.7958) centre (-14.5, 55.2958) ccw projected
  line L11 (-9.2085, 69.2958) -> (-9.2085, 68.7958) projected
  point P0 (0, 0)
  point P1 (-25.5572, 65.2958)
  point P2 (-9.2085, 69.2958)
  point P3 (-9.2085, 69.2958)
  dimension "d34" = 5.2
  dimension "d36" = 1.2
  dimension "d177" = 0.5
  constraints: 8 end point, 2 perpendicular, 1 coincident, 1 vertical, 3 other
  measures "d34" distance edge to line of A121 L7
  measures "d177" distance edge to line of A121 L8
extrude "Extrusion4" add sketch "Sketch3" along normal blind 14.75 contours L6 L5 L4 L3 L2 L1 A121 L11 L0 | L11 A121 L8 | A121 L9 L7 L8 | A121 L7 L8
sketch "Sketch4" plane through (0, 0, -34.5) normal (0, 0, -1) x (-1, 0, 0)
  line L0 (6, 69.2958) -> (6, 90.2856) projected
  line L1 (6, 90.2856) -> (3, 90.8556) projected
  line L2 (3, 90.8556) -> (3, 81.4) projected
  line L3 (3, 81.4) -> (0, 81.4) projected
  line L4 (0, 81.4) -> (0, 65.2958) projected
  line L5 (1.4182, 66.1564) -> (0, 66.2059)
  line L6 (27, 52.5631) -> (27, 86.2958)
  line L7 (27, 86.2958) -> (6, 90.2856)
  line L8 (27, 86.2958) -> (6.5, 86.2958) projected
  circle A0 centre (14.5, 55.2958) radius 14.5 projected
  circle A1 centre (14.5, 55.2958) radius 13.85 projected
  line L9 (26.0532, 65.2961) -> (22.0556, 65.4357) projected
  line L10 (5.4157, 66.0168) -> (22.0556, 65.4357) projected
  line L11 (5.4157, 66.0168) -> (1.4182, 66.1564) projected
  line L12 (-0.1879, 65.2958) -> (27, 65.2958)
  line L13 (26.0531, 65.2961) -> (26.0607, 65.2958)
  line L14 (23.8, 69.2958) -> (6, 69.2958) projected
  line L15 (0, 65.2958) -> (23.8, 65.2958) projected
  line L16 (23.8, 65.2958) -> (23.8, 69.2958) projected
  line L17 (23.8, 65.2958) -> (27, 65.2958)
  line L18 (27, 65.2958) -> (27, 69.2958)
  line L19 (27, 69.2958) -> (23.8, 69.2958)
  line L20 (23.8, 69.2958) -> (23.8, 65.2958)
  point P0 (0, 0)
  point P1 (4.7624, 66.0396)
  point P2 (24.9634, 65.3342)
  point P3 (3, 66.1011)
  point P4 (21.5929, 65.4519)
  point P5 (24.3577, 65.3553)
  point P6 (27, 62.6443)
  point P7 (25, 65.2958)
  point P8 (23.8, 65.3748)
  dimension "d24" = 0
  dimension "d37" = 2
  dimension "d178" = 4.5
  dimension "d179" = 4
  constraints: 18 end point, 7 point on line, 2 collinear, 2 parallel, 2 perpendicular, 1 horizontal, 1 vertical
  measures "d24" distance from line of L6.end L8
  measures "d37" distance edge to line of A0 L6
  measures "d178" distance edge to line of A0 L12
  measures "d179" distance between parallel lines of L12 L19
extrude "Extrusion7" add sketch "Sketch4" along normal blind 15.5 contours L14 A0 L11 L5 L4 L3 L2 L1 L0 | L0 L7 L6 L19 L14 A0 | L14 A0 L16 A1 L10 L11 | A0 L14 | L14 L16 A0 | L6 L12 L9 A0 L16 L19 | A0 L9 A1 L16 | L16 L9 L10 A1 | A1 L9 L16
ref_plane "Work Plane4" through (-23.1368, 52.6716, -30.5) normal (0, 0, 1) x (0.9993908, 0.0348995, 0)
ref_plane "Work Plane8" through (-43.2823, 9.5041, -29.35) normal (0, 0, -1) x (-0.3802684, 0.9248762, 0)
ref_plane "Work Plane9" through (-49.9646, -8.4408, -26.85) normal (0, 0, 1) x (0.9248762, 0.3802684, 0)
extrude "Extrusion8" add sketch "Sketch4" against normal up to surface (7.65 mm away) contours L6 L12 L9 A0 L16 L19 | A0 L9 A1 L16 | L9 L12 A0 | A0 L12 A1 L9 | A1 L9 L16 | A1 L12 L16 L9
ref_plane "Work Plane5" through (-23.1368, 52.6716, -30.5) normal (0, 0, 1) x (0.9993908, 0.0348995, 0)
ref_plane "Work Plane10" through (-43.2823, 9.5041, -29.35) normal (0, 0, -1) x (-0.3802684, 0.9248762, 0)
extrude "Extrusion9" cut sketch "Sketch4" against normal up to surface (5.15 mm away) contours L11 L10 A1 L12 A0 | A0 L12 L4 L5 L11 | L9 L12 A0 | A0 L12 A1 L9 | A1 L10 L9 L16 L12 | A1 L12 L16 L9
ref_plane "Work Plane1" through (-5, 81.9, -49.5) normal (0, 0, -1) x (0, 1, 0)
ref_plane "Work Plane2" through (-13.7612, 65.7253, -40) normal (-0.0348995, 0.9993908, 0) x (-0.9993908, -0.0348995, 0)
ref_plane "Work Plane3" through (-23.8, 0, -27.5) normal (0, 0, -1) x (0, 1, 0)
sketch "Sketch5" plane through (-13.7612, 65.7253, -40) normal (-0.0348995, 0.9993908, 0) x (-0.9993908, -0.0348995, 0)
  arc A0 (0, -0.2709) -> (0, -0.7291) centre (-5.245, -0.5) ccw projected
  arc A1 (0, -0.7291) -> (0, -0.2709) centre (5.245, -0.5) ccw projected
  circle A2 centre (-5.245, -0.5) radius 4.5 projected
  circle A3 centre (5.245, -0.5) radius 4.5 projected
  line L0 (0.5, 1.7467) -> (-0.5, 1.7467)
  line L1 (0.5, -2.7467) -> (-0.5, -2.7467)
  line L2 (0.5, 1.7467) -> (1.346, 1.7467)
  line L3 (-0.5, 1.7467) -> (-1.346, 1.7467)
  line L4 (-0.5, -2.7467) -> (-1.346, -2.7467)
  line L5 (0.5, -2.7467) -> (1.346, -2.7467)
  point P0 (-11.4591, 40)
  dimension "d30" = 1
  dimension "d31" = 1
  constraints: 12 end point, 8 point on circle, 3 point on line, 2 parallel, 1 horizontal
  measures "d30" distance of L0.start L0.end
  measures "d31" distance of L1.start L1.end
extrude "Extrusion14" cut sketch "Sketch5" along normal blind 2.5
extrude "Extrusion15" cut sketch "Sketch5" along normal through all contours A1 L2 A3 L5 A0 L4 A2 L3 | A0 L0 A1 | A0 A1 L1 | A2 | A3
sketch "Sketch8" plane through (-3, 81.4, 34.5) normal (0, 1, 0) x (1, 0, 0)
  line L0 (1.37, 83.5) -> (1.37, 67.5) projected
  line L1 (0.37, 83.5) -> (1.37, 83.5) projected
  line L2 (0.37, 67.5) -> (0.37, 83.5) projected
  line L3 (0.37, 67.5) -> (1.37, 67.5) projected
  line L4 (1.37, 83.5) -> (1.87, 83.5)
  line L5 (1.87, 83.5) -> (1.87, 67)
  line L6 (1.87, 67) -> (0.37, 67)
  line L7 (0.37, 67) -> (0.37, 67.5)
  point P0 (3, 34.5)
  dimension "d54" = 0.5
  dimension "d55" = 0.5
  constraints: 8 end point, 2 perpendicular, 1 horizontal, 1 parallel
  measures "d54" distance between parallel lines of L6 L3
  measures "d55" distance between parallel lines of L5 L0
extrude "Extrusion11" cut sketch "Sketch8" against normal through all
sketch "Sketch9" plane through (-27, 69.2958, -34.5) normal (-1, 0, 0) x (0, 0, 1)
  line L0 (-14.5, -3.0638) -> (1.5, -3.0638) projected
  line L1 (1.5, -3.0638) -> (1.5, 12.9362) projected
  line L2 (1.5, 12.9362) -> (-14.5, 12.9362) projected
  line L3 (-14.5, 12.9362) -> (-14.5, -3.0638) projected
  circle A0 centre (-12.475, 1.0762) radius 0.45 projected
  circle A1 centre (-4, 3.4362) radius 1.25 projected
  circle A2 centre (-12.475, 8.6962) radius 0.45 projected
  circle A3 centre (-12.475, 3.6962) radius 0.45 projected
  circle A4 centre (-12.475, 6.1562) radius 0.45 projected
  line L4 (-11.25, -2.2536) -> (-11.25, 18.535) construction
  line L5 (-14.5, 9.1462) -> (-12.025, 9.1462)
  line L6 (-12.025, 9.1462) -> (-12.025, 0.6262)
  line L7 (-12.025, 0.6262) -> (-14.5, 0.6262)
  line L8 (-14.5, 0.6262) -> (-14.5, 9.1462)
  ellipse E0 centre (-6, -1.8875) end of major axis (-0.75, -1.8875) minor radius 0.1832 (-5.7709, -2.0705) -> (-6.2291, -2.0705) ccw projected
  ellipse E1 centre (-6, -2.2536) end of major axis (-0.75, -2.2536) minor radius 0.1832 (-6.2291, -2.0705) -> (-5.7709, -2.0705) ccw projected
  ellipse E2 centre (-6, -1.8875) end of major axis (-1.5, -1.8875) minor radius 0.157 projected
  ellipse E3 centre (-6, -2.2536) end of major axis (-1.5, -2.2536) minor radius 0.157 projected
  point P0 (34.5, -69.2958)
  point P1 (-13.5, 8.4142)
  point P2 (-13.5, -3.9142)
  dimension "d58" = 0
  dimension "d59" = 0.775
  dimension "d60" = 0
  dimension "d61" = 0
  constraints: 10 end point, 2 parallel, 2 vertical, 1 horizontal, 1 perpendicular, 1 point on line, 3 other
  measures "d58" distance edge to line of A2 L6
  measures "d59" distance between parallel lines of L4 L6
  measures "d60" distance edge to line of A2 L5
  measures "d61" distance edge to line of A0 L7
extrude "Extrusion12" cut sketch "Sketch9" against normal up to surface (25.87 mm away) contours A3 | A4 | L3 L5 A2 L6 A0 L7 | A0 | A0 L6 L7 | L5 L6 A2 | A2
fillet "Fillet1" radius 2 3 edges at (-2.63, 74.182, -46.525) (-2.63, 78.442, -47.7625) (-2.63, 69.922, -47.7625)
sketch "Sketch10" plane through (0, 65.2958, 34.5) normal (1, 0, 0) x (0, 0, -1)
  line L0 (80.4, 14.1042) -> (80.4, 3.5362)
  line L1 (80.4, 3.5362) -> (75.9, 3.5362)
  line L2 (75.9, 3.5362) -> (75.9, 14.1042)
  line L3 (75.9, 14.1042) -> (75.9, 16.9362)
  line L4 (80.4, 16.9362) -> (80.4, 14.1042)
  line L5 (67.5, 16.9362) -> (67.5, 0.9362) projected
  line L6 (67.5, 0.9362) -> (83.5, 0.9362) projected
  line L7 (83.5, 0.9362) -> (83.5, 16.9362) projected
  line L8 (83.5, 16.9362) -> (67.5, 16.9362) projected
  line L9 (79.9, 13.8362) -> (79.9, 10.3362) projected
  line L10 (79.9, 10.3362) -> (76.4, 10.3362) projected
  line L11 (76.4, 10.3362) -> (76.4, 13.8362) projected
  line L12 (76.4, 13.8362) -> (79.9, 13.8362) projected
  line L13 (76.4, 7.5362) -> (79.9, 7.5362) projected
  line L14 (79.9, 7.5362) -> (79.9, 4.0362) projected
  line L15 (79.9, 4.0362) -> (76.4, 4.0362) projected
  line L16 (76.4, 4.0362) -> (76.4, 7.5362) projected
  circle A0 centre (81.475, 5.0762) radius 0.45 projected
  circle A1 centre (73, 7.4362) radius 1.25 projected
  circle A2 centre (81.475, 12.6962) radius 0.45 projected
  circle A3 centre (81.475, 7.6962) radius 0.45 projected
  circle A4 centre (81.475, 10.1562) radius 0.45 projected
  point P0 (34.5, -65.2958)
  dimension "d151" = 0.5
  dimension "d152" = 0.5
  dimension "d153" = 0.5
  constraints: 10 end point, 2 point on line, 1 collinear, 1 parallel
  measures "d151" distance between parallel lines of L9 L0
  measures "d152" distance between parallel lines of L2 L11
  measures "d153" distance between parallel lines of L1 L15
extrude "Extrusion13" cut sketch "Sketch10" against normal up to surface (1.13 mm away) contours L0 L1 L2 L3 L8 L4 | L9 L10 L11 L12 | L13 L14 L15 L16
ref_plane "Work Plane6" through (-13.7612, 65.7253, -40) normal (-0.0348995, 0.9993908, 0) x (-0.9993908, -0.0348995, 0)
sketch "Sketch12" plane through (-13.7612, 65.7253, -40) normal (-0.0348995, 0.9993908, 0) x (-0.9993908, -0.0348995, 0)
  circle A0 centre (9.5744, 6.0491) radius 0.75 projected
  circle A1 centre (-0.0256, -6.5) radius 0.75 projected
  circle A2 centre (-9.6256, 6.0491) radius 0.75 projected
  point P0 (-11.4591, 40)
hole "Hole2" at (-23.3298, 65.3912, -33.9509) at (-13.7357, 65.7262, -46.5) at (-4.1415, 66.0613, -33.9509) direction (-0.0348995, 0.9993908, 0) diameter 2.5 depth 5 counterbore diameter 3 counterbore depth 1
sketch "Sketch16" plane through (-27, 69.2958, -34.5) normal (-1, 0, 0) x (0, 0, 1)
  line L0 (-12.025, 9.1462) -> (-12.025, 0.6262) projected
  line L1 (-15.5, -4) -> (-15.5, 17) projected
  line L2 (-12.025, 8.4142) -> (0, 8.5)
  line L3 (-13.25, 0.6262) -> (-12.025, 0.6262) projected
  line L4 (-1.5, -0.889) -> (-1.5, 20.3536) projected
  line L5 (-12.025, 0.6262) -> (-10.025, -1.3738) projected
  line L6 (0, 0) -> (-12.025, 0.6262)
  line L7 (0, 0) -> (0, 17) projected
  line L8 (0, 17) -> (-15.5, 17) projected
  line L9 (7.65, -4) -> (-15.5, -4) projected
  line L10 (7.65, -4) -> (7.65, 0) projected
  line L11 (0, 0) -> (7.65, 0) projected
  point P0 (34.5, -69.2958)
  point P1 (-11.025, -0.1058)
  point P2 (-1.5, 8.4893)
  point P3 (-12.025, 8.4142)
  point P4 (-12.025, -0.1058)
  point P5 (0, 8.5)
  constraints: 4 end point, 2 other
extrude "Extrusion16" cut sketch "Sketch16" against normal blind 2 contours L2 L4 L6 L0 | L2 L7 L6 L4